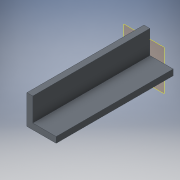
# Autodesk Inventor part: inside Angle beam
Saved by Autodesk Inventor 2016 (Build 200138000, 138)
## iProperties
Created: 2015-08-29
Part Number: inside Angle beam
Material: Generic
Description: ANGLE - 144 MM
Document SubType Name: Modeling
Designer: PTC
Density: 1 g/cm^3
Appearance: Default
Sending System: Creo  TM  2.0  (c) 2012
PROJECT: FTC
PTC_MATERIAL_NAME: METAL_ALUMINIUM_5052
NIKCONFIGCOUNT: 1
KIT: TETRIX
Author: phi
Autodesk Inventor part; units mm, degrees
ref_plane "YZ Plane" through (0, 0, 0) normal (1, 0, 0) x (0, 1, 0)
ref_plane "XZ Plane" through (0, 0, 0) normal (0, 1, 0) x (-1, 0, 0)
ref_plane "XY Plane" through (0, 0, 0) normal (0, 0, 1) x (1, 0, 0)
ref_plane "FRONT" through (0, 0, 0) normal (0, 0, 1) x (1, 0, 0)
ref_plane "TOP" through (0, 0, 0) normal (0, 1, 0) x (-1, 0, 0)
ref_plane "RIGHT" through (0, 0, 0) normal (1, 0, 0) x (0, 1, 0)
ref_plane "Work Plane4" through (0, 0, 0) normal (0, 0, 1) x (1, 0, 0)
sketch "Sketch1" plane through (0, 0, 0) normal (0, 0, 1) x (1, 0, 0)
  line L0 (3.2, 16) -> (0, 16) projected
  line L1 (3.2, 3.2) -> (3.2, 14) projected
  line L2 (3.2, 14) -> (3.2, 16) projected
  line L3 (0, 16) -> (0, 14) projected
  line L4 (0, 14) -> (0, 0) projected
  line L5 (0, 0) -> (14, 0) projected
  line L6 (16, 0) -> (16, 3.2) projected
  line L7 (16, 3.2) -> (14, 3.2) projected
  line L8 (14, 3.2) -> (3.2, 3.2) projected
  line L9 (14, 0) -> (16, 0) projected
extrude "Extrusion1" add sketch "Sketch1" along normal blind 64
body "Solid2"
